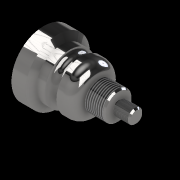
# Autodesk Inventor part: Tarefa 2
Saved by Autodesk Inventor 2020 (Build 240168000, 168)
## iProperties
Created: 2020-12-15
Part Number: Tarefa 2
Material: Bronze, Cast
Document SubType Name: Modeling
Designer: Mr Random
Density: 8.87 g/cm^3
Appearance: Steel - Polished
Author: Mr Random
Autodesk Inventor part; units mm, degrees
ref_plane "YZ Plane" through (0, 0, 0) normal (1, 0, 0) x (0, 1, 0)
ref_plane "XZ Plane" through (0, 0, 0) normal (0, 1, 0) x (-1, 0, 0)
ref_plane "XY Plane" through (0, 0, 0) normal (0, 0, 1) x (1, 0, 0)
sketch "Sketch1" plane through (0, 0, 0) normal (0, 0, 1) x (1, 0, 0)
  line L0 (0, 0) -> (20, 0)
  line L1 (20, 35) -> (20, 45)
  line L2 (20, 45) -> (0, 45)
  line L3 (0, 45) -> (0, 0)
  line L4 (20, 0) -> (25, 0)
  line L5 (25, 0) -> (25, 35)
  line L6 (20, 35) -> (20, 0)
  line L7 (25, 0) -> (37, 0)
  line L8 (37, 0) -> (37, 35)
  line L9 (37, 35) -> (25, 35)
  line L10 (25, 35) -> (25, 0)
  line L11 (20, 45) -> (25, 35)
  line L12 (37, 0) -> (53, 0)
  line L13 (53, 0) -> (53, 35)
  line L14 (37, 35) -> (37, 0)
  arc A0 (37, 35) -> (53, 35) centre (45, 35) ccw
  line L15 (53, 0) -> (75, 0)
  line L16 (75, 0) -> (75, 20)
  line L17 (60, 35) -> (53, 35)
  line L18 (53, 35) -> (53, 0)
  arc A1 (75, 20) -> (60, 35) centre (60, 20) ccw
  arc A2 (53, 33.2665) -> (52.7831, 33.1498) centre (60, 20) ccw
  line L19 (75, 0) -> (78, 0)
  line L20 (78, 0) -> (78, 15)
  line L21 (78, 15) -> (75, 15)
  line L22 (75, 15) -> (75, 0)
  line L23 (78, 0) -> (105, 0)
  line L24 (105, 0) -> (105, 20)
  line L25 (105, 20) -> (78, 20)
  line L26 (78, 20) -> (78, 0)
  line L27 (105, 0) -> (108, 0)
  line L28 (108, 0) -> (108, 7.5)
  line L29 (108, 7.5) -> (105, 7.5)
  line L30 (105, 7.5) -> (105, 0)
  line L31 (108, 0) -> (130, 0)
  line L32 (130, 0) -> (130, 10)
  line L33 (130, 10) -> (108, 10)
  line L34 (108, 10) -> (108, 0)
  line L35 (164.0679, 0) -> (-30.9325, 0)
  line L36 (-30.9325, 35) -> (60, 35)
  line L37 (75, 35) -> (164.0679, 35)
  line L38 (60, 35) -> (75, 35)
  point P0 (53, 33.2665)
  dimension "d0" = 20
  dimension "d4" = 12
  dimension "d5" = 35
  dimension "d7" = 16
  dimension "d9" = 22
  dimension "d12" = 3
  dimension "d13" = 15
  dimension "d14" = 27
  dimension "d15" = 20
  dimension "d16" = 3
  dimension "d17" = 7.5
  dimension "d18" = 22
  dimension "d19" = 10
  dimension "d20" = 45
  dimension "d21" = 5
  dimension "d22" = 15
  dimension "d23" = 7
  constraints: 78 end point, 16 parallel, 12 horizontal, 9 perpendicular, 7 point on circle, 4 point on line, 4 tangent, 3 centre point, 1 coincident
  measures "d0" distance of L2.end L1.end
  measures "d4" distance of L9.end L8.end
  measures "d5" distance of L8.end L7.end
  measures "d7" distance of L14.start L13.end
  measures "d9" distance of L17.end L37.start
  measures "d12" distance of L21.end L20.end
  measures "d13" distance of L20.end L19.end
  measures "d14" distance of L25.end L24.end
  measures "d15" distance of L23.end L24.end
  measures "d16" distance of L29.end L28.end
  measures "d17" distance of L28.end L27.end
  measures "d18" distance of L33.end L32.end
  measures "d19" distance of L32.end L31.end
  measures "d20" distance of L2.end L0.start
  measures "d21" horizontal distance of L1.end L9.end
  measures "d22" radius of A1
  measures "d23" distance of L13.end L17.start
revolve "Revolution1" add sketch "Sketch1" angle 360 about axis through (164.0679, 0, 0) along (-1, 0, 0) contours L3 L36 L6 L0 | L6 L36 L5 L4 | L3 L2 L1 L36 | L5 L9 L8 L7 | L1 L11 L36 | L8 A0 A2 L13 L12 | L13 L17 A1 L16 L15 | L16 L21 L20 L19 | L20 L26 L25 L24 L23 | L24 L29 L28 L27 | L28 L34 L33 L32 L31
chamfer "Chamfer1" distance 2 angle 45 1 edges at (105, -20, 0)
chamfer "Chamfer2" distance 2 angle 45 1 edges at (130, -10, 0)
thread "Thread1" size "M40x3" class "6g" standard "ANSI Metric M Profile" full length
thread "Thread2" size "M20x1" class "6g" standard "ANSI Metric M Profile" full length
body "Solid1"
